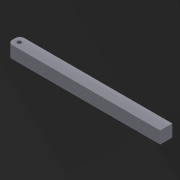
# Autodesk Inventor part: virsutinis
Saved by Autodesk Inventor 2019 (Build 230136000, 136)
## iProperties
Created: 2014-11-18
Part Number: virsutinis
Material: Stainless Steel AISI 440C, Welded
Document SubType Name: Modeling
Designer: Ben
Density: 7.8 g/cm^3
Appearance: Weld - Stainless Steel
Mass: 2012.63 g
Surface Area: 1247.9 cm^2
Volume: 249.088 cm^3
Author: Ben
Autodesk Inventor part; units mm, degrees
ref_plane "YZ Plane" through (0, 0, 0) normal (1, 0, 0) x (0, 1, 0)
ref_plane "XZ Plane" through (0, 0, 0) normal (0, 1, 0) x (-1, 0, 0)
ref_plane "XY Plane" through (0, 0, 0) normal (0, 0, 1) x (1, 0, 0)
sketch "Sketch1" plane through (0, 0, 0) normal (0, 0, 1) x (1, 0, 0)
  circle A0 centre (0, 0) radius 6
  line L0 (-18, 20) -> (482, 20)
  line L1 (482, -20) -> (-18, -20)
  line L2 (-18, -5) -> (-18, 5)
  arc A1 (-3, 20) -> (-18, 5) centre (-3, 5) ccw
  arc A2 (-18, -5) -> (-3, -20) centre (-3, -5) ccw
  line L3 (482, 0) -> (482, 0)
  line L4 (482, -20) -> (482, 20)
  dimension "d0" = 12
  dimension "d3" = 18
  dimension "d5" = 40
  dimension "d6" = 20
  dimension "d7" = 15
  dimension "d36" = 500
  constraints: 11 end point, 5 point on line, 4 point on circle, 4 tangent, 3 centre point, 2 parallel, 2 vertical, 1 coincident, 1 equal radius, 1 horizontal
  measures "d0" diameter of A0
  measures "d3" distance from line of L2 point (0, 0)
  measures "d5" distance between parallel lines of L1 L0
  measures "d6" distance from line of L0 A0.centre
  measures "d7" radius of A1
  measures "d36" distance between parallel lines of L4 L2
extrude "Extrusion1" add sketch "Sketch1" along normal blind 40
ref_plane "Work Plane1" through (0, 0, 20) normal (0, 0, 1) x (1, 0, 0)
chamfer "Chamfer1" distance 1 angle 45 2 edges at (-6, 0, 0) (-6, 0, 40)
shell "Shell2" thickness 5 removed faces 1 at (482, -6.6667, 26.6667)
sketch "Sketch7" plane through (-3, -20, 0) normal (0, -1, 0) x (1, 0, 0)
  line L0 (35, 35) -> (-15, 35)
  line L1 (-15, 35) -> (-15, 5)
  line L2 (-15, 5) -> (35, 5)
  line L3 (35, 5) -> (35, 35)
  line L4 (35, 35) -> (-15, 5) construction
  line L5 (-15, 35) -> (35, 5) construction
  line L6 (-15, 0) -> (-15, 40) projected
  line L7 (-15, 20) -> (35, 20)
  dimension "d38" = 30
  dimension "d40" = 50
  constraints: 14 end point, 3 parallel, 2 perpendicular, 1 midpoint, 1 point on line, 1 vertical, 1 other
  measures "d38" distance of L1.end L0.end
  measures "d40" distance of L0.start L0.end
extrude "Extrusion7" cut sketch "Sketch7" against normal through all
body "Solid1"
